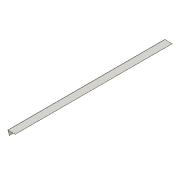
# Autodesk Inventor part: Angle--Back
Saved by Autodesk Inventor 2018 (Build 220112000, 112)
## iProperties
Created: 2017-07-14
Part Number: Angle--Back
Material: Generic
Document SubType Name: Modeling
Designer: thoma
Density: 1 g/cm^3
Appearance: Steel
Author: thoma
Autodesk Inventor part; units mm, degrees
ref_plane "YZ Plane" through (0, 0, 0) normal (1, 0, 0) x (0, 1, 0)
ref_plane "XZ Plane" through (0, 0, 0) normal (0, 1, 0) x (-1, 0, 0)
ref_plane "XY Plane" through (0, 0, 0) normal (0, 0, 1) x (1, 0, 0)
sketch "Sketch1" plane through (0, 0, 0) normal (0, 0, 1) x (1, 0, 0)
  line L0 (-1.8974, -23.3494) -> (-1.8974, -74.3026)
  line L1 (-1.8974, -74.3026) -> (0, -74.3026)
  line L2 (0, -74.3026) -> (0, 0)
  line L3 (0, 0) -> (99.7026, 0)
  line L4 (99.7026, 0) -> (99.7026, 1.8974)
  line L5 (99.7026, 1.8974) -> (-1.8974, 1.8974)
  line L6 (-1.8974, 1.8974) -> (-1.8974, -23.3494)
  dimension "d0" = 101.6
  dimension "d1" = 76.2
  dimension "d2" = 1.8974
  dimension "d3" = 1.8974
  constraints: 14 end point, 3 parallel, 1 horizontal, 1 perpendicular
  measures "d0" distance of L4.end L5.end
  measures "d1" distance of L0.end L5.end
  measures "d2" distance of L0.end L1.end
  measures "d3" distance of L3.end L4.end
extrude "Extrusion1" add sketch "Sketch1" against normal blind 2159
sketch "Sketch2" plane through (0, -74.3026, 0) normal (1, 0, 0) x (0, 0, -1)
  line L0 (0, 74.3026) -> (19.9093, 0)
  line L1 (0, 0) -> (2159, 0) projected
  line L2 (19.9093, 0) -> (0, 0)
  line L3 (0, 0) -> (0, 74.3026)
  dimension "d6" = 15
  constraints: 6 end point, 2 point on line, 1 horizontal, 1 perpendicular
  measures "d6" angle of L3 L0
extrude "Extrusion2" cut sketch "Sketch2" against normal up to next
body "Solid1"
